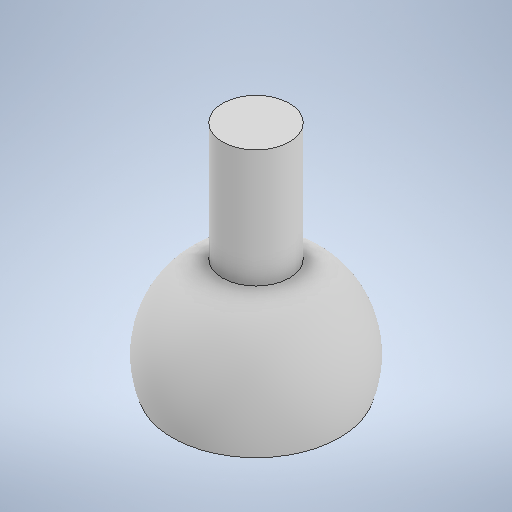
# Autodesk Inventor part: DummyBallJointF
Saved by Autodesk Inventor 2025.2 (Build 292293000, 293)
## iProperties
Created: 2025-01-08
Part Number: DummyBallJointF
Material: 일반
Document SubType Name: Modeling
Designer: SEON
Density: 1 g/cm^3
Appearance: 기본값
Author: SEON
Autodesk Inventor part; units mm, degrees
ref_plane "YZ Plane" through (0, 0, 0) normal (1, 0, 0) x (0, 1, 0)
ref_plane "XY Plane" through (0, 0, 0) normal (0, 0, 1) x (1, 0, 0)
sketch "스케치1" plane through (0, 0, 0) normal (0, 0, 1) x (1, 0, 0)
  circle A0 centre (0, 0) radius 2.5
  circle A1 centre (0, 0) radius 4
  line L0 (0, 4) -> (0, -4)
  line L1 (0, 0) -> (-3.7588, -1.3681)
  point P0 (-2.3492, -0.8551)
  point P1 (0, 2.5)
  dimension "d0" = 5
  dimension "d1" = 1.5
  dimension "d2" = 110
  constraints: 4 end point, 3 point on circle, 2 centre point, 1 coincident, 1 midpoint, 1 vertical
  measures "d0" diameter of A0
  measures "d1" radial gap between concentric circles of A0 A1
  measures "d2" angle of L0 L1
revolve "회전1" add sketch "스케치1" angle 360 about axis through (0, 4, 0) along (0, -1, 0) picked at (-3.3614, -0.8862) contours A0 L1 A1 L0
ref_plane "작업 평면1" through (0, 4, 0) normal (0, 1, 0) x (-1, 0, 0)
sketch "스케치2" plane through (0, 4, 0) normal (0, 1, 0) x (-1, 0, 0)
  circle A0 centre (0, 0) radius 1.5
  dimension "d4" = 3
  constraints: 1 centre point, 1 coincident
  measures "d4" diameter of A0
extrude "돌출1" add sketch "스케치2" along normal blind 5 and the other way blind 1
